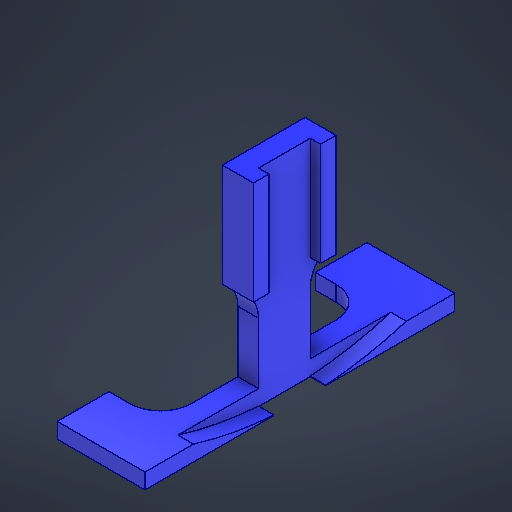
# Autodesk Inventor part: measuring_disk_stander
Saved by Autodesk Inventor 2026.1 (Build 301233000, 233)
## iProperties
Created: 2025-12-30
Part Number: measuring_disk_stander
Material: Generic
Document SubType Name: Modeling
Designer: emanuel
Density: 1 g/cm^3
Appearance: Blue - Wall Paint - Glossy
Author: emanuel
Autodesk Inventor part; units mm, degrees
ref_plane "YZ Plane" through (0, 0, 0) normal (1, 0, 0) x (0, 1, 0)
ref_plane "XZ Plane" through (0, 0, 0) normal (0, 1, 0) x (-1, 0, 0)
ref_plane "XY Plane" through (0, 0, 0) normal (0, 0, 1) x (1, 0, 0)
sketch "Sketch1" plane through (0, 0, 0) normal (1, 0, 0) x (0, 1, 0)
  circle A0 centre (0, 0) radius 70
  line L0 (-70, 0) -> (-70, -30)
  line L1 (-70, -30) -> (-70, 30)
  line L2 (-70, 30) -> (-67, 30)
  line L3 (-67, 30) -> (-67, -30)
  line L4 (-67, -30) -> (-70, -30)
  line L5 (-70, 0) -> (-70, -5)
  line L6 (-70, -5) -> (-30, -5)
  line L7 (-30, -5) -> (-30, 5)
  line L8 (-30, 5) -> (-70, 5)
  line L9 (-70, 5) -> (-70, -5)
  point P0 (-67, -20.2731)
  point P1 (-69.8212, -5)
  point P2 (-69.8212, 5)
  point P3 (-67, 20.2731)
  point P4 (-67, 5)
  point P5 (-67, -5)
  dimension "d0" = 140
  dimension "d1" = 30
  dimension "d2" = 60
  dimension "d3" = 3
  dimension "d4" = 5
  dimension "d5" = 40
  dimension "d6" = 10
  constraints: 20 end point, 4 perpendicular, 2 parallel, 2 point on line, 2 vertical, 1 coincident, 1 horizontal, 3 other
  measures "d1" distance of L0.start L0.end
  measures "d2" distance of L0.end L1.end
  measures "d3" distance of L1.end L2.end
  measures "d4" distance of L0.start L5.end
  measures "d5" distance of L8.end L7.end
  measures "d6" distance of L7.end L6.end
extrude "Extrusion1" add sketch "Sketch1" along normal blind 3 contours A0 L8 L1 L2 L3 | L3 L4 L0 L6 A0
extrude "Extrusion2" add sketch "Sketch1" against normal blind 4 contours L3 L8 A0 | A0 L8 L1 L2 L3 | L3 L4 L0 L6 A0 | A0 L6 L3 | L8 L3 L6 A0 | A0 L1 L8 | L8 L7 L6 L3 | L6 L0 A0
sketch "Sketch2" plane through (-4, 0, 0) normal (-1, 0, 0) x (0, 0, 1)
  line L0 (-30, -67) -> (-30, -70) projected
  line L1 (-30, -70) -> (30, -70) projected
  line L2 (-30, -67) -> (-20, -67)
  line L3 (-20, -67) -> (-20, -70)
  line L4 (-20, -70) -> (-30, -70)
  line L5 (-30, -70) -> (-30, -67)
  line L6 (30, -67) -> (20, -67)
  line L7 (20, -67) -> (20, -70.1551)
  line L8 (20, -70.1551) -> (30, -70.1551)
  line L9 (30, -70.1551) -> (30, -67)
  point P0 (0, 0)
  point P1 (20, -70)
  dimension "d11" = 10
  dimension "d12" = 10
  constraints: 16 end point, 4 parallel, 2 horizontal, 2 perpendicular, 2 point on line
  measures "d11" distance of L3.end L4.end
  measures "d12" distance of L8.end L7.end
extrude "Extrusion3" add sketch "Sketch2" along normal blind 10 contours L2 L3 L1 L0 | L7 L6 L9 L1
fillet "Fillet1" radius 6 2 edges at (-4, -68.5, -20) (-4, -68.5, 20)
sketch "Sketch3" plane through (3, 0, 0) normal (1, 0, 0) x (0, 0, -1)
  arc A0 (-20.2731, -67) -> (-5, -69.8212) centre (0, 0) ccw projected
  circle A1 centre (0, 0) radius 70.1
  circle A2 centre (0, 0) radius 70
  point P0 (-5, -69.8212)
  dimension "d16" = 140.2
  dimension "d17" = 140
  constraints: 2 centre point, 2 coincident
  measures "d16" diameter of A1
  measures "d17" diameter of A2
extrude "Extrusion4" cut sketch "Sketch3" against normal blind 3
sketch "Sketch4" plane through (0, -30, 5) normal (0, 1, 0) x (1, 0, 0)
  line L0 (-4, 0) -> (2, 0)
  line L1 (2, 0) -> (2, -3)
  line L2 (2, -3) -> (-4, -3)
  line L3 (-4, -3) -> (-4, 0)
  line L4 (0, 10) -> (-4, 10) projected
  line L5 (-4, 10) -> (2, 10)
  line L6 (2, 10) -> (2, 13)
  line L7 (2, 13) -> (-4, 13)
  line L8 (-4, 13) -> (-4, 10)
  point P0 (0, 5)
  dimension "d20" = 6
  dimension "d21" = 3
  dimension "d22" = 6
  dimension "d23" = 3
  constraints: 16 end point, 4 parallel, 2 horizontal, 2 perpendicular
  measures "d20" distance of L1.end L2.end
  measures "d21" distance of L0.end L1.end
  measures "d22" distance of L7.end L6.end
  measures "d23" distance of L6.end L5.end
extrude "Extrusion5" add sketch "Sketch4" against normal blind 20
fillet "Fillet2" radius 6 2 edges at (-2, -50, 5) (-2, -50, -5)
body "Solid1"
